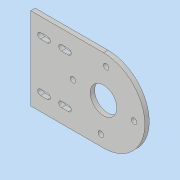
# Autodesk Inventor part: MMplate2
Saved by Autodesk Inventor 2017 (Build 210142000, 142)
## iProperties
Created: 2016-12-23
Part Number: MMplate2
Material: Generic
Document SubType Name: Modeling
Designer: Joshua Yuan
Density: 1 g/cm^3
Appearance: Default
Author: Joshua Yuan
Autodesk Inventor part; units mm, degrees
note: some values were not read from the file. Chosen so that the rebuilt part matches the saved one: sketch regions of "Extrusion1".
ref_plane "YZ Plane" through (0, 0, 0) normal (1, 0, 0) x (0, 1, 0)
ref_plane "XZ Plane" through (0, 0, 0) normal (0, 1, 0) x (-1, 0, 0)
ref_plane "XY Plane" through (0, 0, 0) normal (0, 0, 1) x (1, 0, 0)
sketch "Sketch1" plane through (0, 0, 0) normal (0, 0, 1) x (1, 0, 0)
  circle A0 centre (167.1084, 53.7786) radius 29.5
  line L0 (167.1084, 83.2786) -> (115.1084, 83.2786)
  line L1 (115.1084, 83.2786) -> (115.1084, 24.2786)
  line L2 (115.1084, 24.2786) -> (167.1084, 24.2786)
  circle A1 centre (167.1084, 53.7786) radius 9.525
  circle A2 centre (145.2715, 55.689) radius 2
  circle A3 centre (169.0189, 75.6154) radius 2
  circle A4 centre (188.9453, 51.8681) radius 2
  circle A5 centre (165.1979, 31.9417) radius 2
  line L3 (169.0189, 75.6154) -> (165.1979, 31.9417) construction
  line L4 (188.9453, 51.8681) -> (145.2715, 55.689) construction
  line L5 (-39.3217, 0) -> (235.9301, 0) projected
  line L6 (0, -16.6557) -> (0, 99.9343) projected
  line L7 (167.1084, 53.7786) -> (100.0684, 53.7786) construction
  circle A6 centre (122.0877, 71.2786) radius 2.0193
  circle A7 centre (127.0877, 71.2786) radius 2.0193
  circle A8 centre (137.0877, 71.2786) radius 2.0193
  circle A9 centre (142.0877, 71.2786) radius 2.0193
  circle A10 centre (127.0877, 36.2786) radius 2.0193
  circle A11 centre (122.0877, 36.2786) radius 2.0193
  circle A12 centre (142.0877, 36.2786) radius 2.0193
  circle A13 centre (137.0877, 36.2786) radius 2.0193
  line L8 (127.0877, 73.2979) -> (122.0877, 73.2979)
  line L9 (122.0877, 69.2593) -> (127.0877, 69.2593)
  line L10 (137.0877, 73.2979) -> (142.0877, 73.2979)
  line L11 (142.0877, 69.2593) -> (137.0877, 69.2593)
  line L12 (142.0877, 38.2979) -> (137.0877, 38.2979)
  line L13 (137.0877, 34.2593) -> (142.0877, 34.2593)
  line L14 (127.0877, 38.2979) -> (122.0877, 38.2979)
  line L15 (122.0877, 34.2593) -> (127.0877, 34.2593)
  circle A14 centre (125.0684, 71.2786) radius 2.0193 construction
  circle A15 centre (125.0684, 36.2786) radius 2.0193 construction
  line L16 (125.0684, 71.2786) -> (125.0684, 36.2786) construction
  circle A16 centre (140.0684, 36.2786) radius 2.0193 construction
  circle A17 centre (140.0684, 71.2786) radius 2.0193 construction
  line L17 (140.0684, 71.2786) -> (140.0684, 36.2786) construction
  point P0 (0, 0)
  dimension "d0" = 59
  dimension "d1" = 52
  dimension "d2" = 19.05
  dimension "d3" = 4
  dimension "d4" = 4
  dimension "d5" = 4
  dimension "d6" = 4
  dimension "d7" = 355
  dimension "d8" = 31
  dimension "d9" = 31
  dimension "d10" = 31
  dimension "d11" = 67.04
  dimension "d13" = 4.0386
  dimension "d14" = 4.0386
  dimension "d16" = 4.0386
  dimension "d17" = 4.0386
  dimension "d18" = 4.0386
  dimension "d19" = 4.0386
  dimension "d20" = 4.0386
  dimension "d21" = 4.0386
  dimension "d22" = 5
  dimension "d23" = 5
  dimension "d24" = 5
  dimension "d25" = 5
  dimension "d26" = 4.0386
  dimension "d27" = 25
  dimension "d29" = 15
  dimension "d32" = 35
  constraints: 32 end point, 22 point on circle, 22 tangent, 18 centre point, 6 horizontal, 4 symmetric about line, 3 coincident, 3 perpendicular, 2 equal length, 2 midpoint, 2 vertical, 1 parallel
  measures "d0" diameter of A0
  measures "d1" distance of L0.start L0.end
  measures "d2" diameter of A1
  measures "d3" diameter of A2
  measures "d4" diameter of A3
  measures "d5" diameter of A4
  measures "d6" diameter of A5
  measures "d8" distance of L3.end L4.start
  measures "d9" distance of L4.end L3.end
  measures "d10" distance of L3.start L4.start
  measures "d11" distance of L7.start L7.end
  measures "d13" diameter of A6
  measures "d14" diameter of A7
  measures "d16" diameter of A8
  measures "d17" diameter of A9
  measures "d18" diameter of A10
  measures "d19" diameter of A11
  measures "d20" diameter of A12
  measures "d21" diameter of A13
  measures "d22" distance of A6.centre A7.centre
  measures "d23" distance of A9.centre A8.centre
  measures "d24" distance of A12.centre A13.centre
  measures "d25" distance of A11.centre A10.centre
  measures "d26" diameter of A14
  measures "d27" distance from line of point (100.068, 53.779) L16
  measures "d29" distance between parallel lines of L17 L16
  measures "d32" distance of L16.start L16.end
extrude "Extrusion1" add sketch "Sketch1" along normal blind 3.175 contours A0 A12 A9 | A0 A9 L10 A8 L11 L12 A13 L13 A12 L2 L1 L0
body "Solid1"
